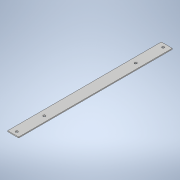
# Autodesk Inventor part: Seat tabsnew
Saved by Autodesk Inventor 2021 (Build 250183000, 183)
## iProperties
Created: 2019-10-29
Part Number: Seat tabsnew
Material: Generic
Document SubType Name: Modeling
Designer: fagang
Density: 1 g/cm^3
Appearance: Default
Description: Seat tabs
Material_size: 1/8" thick steel
Quantity: 2
Author: fagang
Autodesk Inventor part; units mm, degrees
ref_plane "YZ Plane" through (0, 0, 0) normal (1, 0, 0) x (0, 1, 0)
ref_plane "XZ Plane" through (0, 0, 0) normal (0, 1, 0) x (-1, 0, 0)
ref_plane "XY Plane" through (0, 0, 0) normal (0, 0, 1) x (1, 0, 0)
sketch "Sketch1" plane through (0, 0, 0) normal (0, 1, 0) x (-1, 0, 0)
  line L0 (3.9935, 70.1419) -> (-34.1065, 70.1419)
  line L1 (-34.1065, 70.1419) -> (-34.1065, -463.2581)
  line L2 (-34.1065, -463.2581) -> (3.9935, -463.2581)
  line L3 (3.9935, -463.2581) -> (3.9935, 70.1419)
  point P0 (0, 0)
  dimension "d0" = 38.1
  dimension "d1" = 533.4
  constraints: 8 end point, 2 parallel, 1 horizontal, 1 perpendicular
  measures "d0" distance of L2.end L1.end
  measures "d1" distance of L1.end L0.end
extrude "Extrusion1" add sketch "Sketch1" along normal blind 3.175
sketch "Sketch2" plane through (0, 3.175, 0) normal (0, 1, 0) x (1, 0, 0)
  line L0 (-3.9935, -70.1419) -> (34.1065, -70.1419) projected
  circle A0 centre (15.0565, -57.4419) radius 3.9688
  line L1 (34.1065, 463.2581) -> (-3.9935, 463.2581) projected
  circle A1 centre (15.0565, 450.5581) radius 3.9688
  line L2 (34.1065, -70.1419) -> (34.1065, 463.2581) projected
  line L3 (34.1065, 196.5581) -> (-3.9935, 196.5581)
  circle A2 centre (15.0565, 355.3081) radius 3.9688
  circle A3 centre (15.0565, 37.8081) radius 3.9688
  point P0 (0, 0)
  dimension "d5" = 7.9375
  dimension "d7" = 7.9375
  dimension "d10" = 7.9375
  dimension "d11" = 7.9375
  dimension "d14" = 12.7
  dimension "d15" = 107.95
  dimension "d16" = 12.7
  dimension "d17" = 107.95
  constraints: 4 centre point, 2 end point, 1 horizontal, 1 midpoint
  measures "d5" diameter of A0
  measures "d7" diameter of A1
  measures "d10" diameter of A2
  measures "d11" diameter of A3
  measures "d14" distance from line of L0 A0.centre
  measures "d15" distance from line of L0 A3.centre
  measures "d16" distance from line of L1 A1.centre
  measures "d17" distance from line of L1 A2.centre
extrude "Extrusion2" cut sketch "Sketch2" against normal blind 25.4
body "Solid1"
